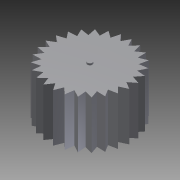
# Autodesk Inventor part: launcher.motor.lowgear
Saved by Autodesk Inventor 2011 (Build 150239000, 239)
## iProperties
Created: 2011-04-05
Part Number: launcher.motor.lowgear
Document SubType Name: Modeling
Designer: Rob
Density: 1 g/cm^3
Author: Rob
Autodesk Inventor part; units mm, degrees
ref_plane "YZ Plane" through (0, 0, 0) normal (1, 0, 0) x (0, 1, 0)
ref_plane "XZ Plane" through (0, 0, 0) normal (0, 1, 0) x (-1, 0, 0)
ref_plane "XY Plane" through (0, 0, 0) normal (0, 0, 1) x (1, 0, 0)
sketch "Sketch1" plane through (0, 0, 0) normal (0, 0, 1) x (1, 0, 0)
  circle A0 centre (0, 0) radius 2
  dimension "d0" = 4
  constraints: 1 centre point, 1 coincident
  measures "d0" diameter of A0
extrude "Extrusion1" add sketch "Sketch1" along normal blind 2.8
sketch "Sketch2" plane through (0, 0, 2.8) normal (0, 0, 1) x (1, 0, 0)
  circle A0 centre (0, 0) radius 0.5
  circle A1 centre (0, 0) radius 2
  line L0 (0, 0) -> (0, 5.155)
  line L1 (0, 2.4402) -> (-0.2438, 1.9851)
  line L2 (0, 2.4402) -> (0.2438, 1.9851)
  arc A2 (0.2438, 1.9851) -> (-0.2438, 1.9851) centre (0, 0) ccw
  line L3 (-0.2438, 1.9851) -> (0, 2.4402)
  line L4 (0, 2.4402) -> (0.2438, 1.9851)
  line L5 (-0.5628, 2.3745) -> (-0.695, 1.8754)
  line L6 (-0.5628, 2.3745) -> (-0.2206, 1.9878)
  arc A3 (-0.2206, 1.9878) -> (-0.695, 1.8754) centre (0, 0) ccw
  line L7 (-1.0952, 2.1807) -> (-1.1087, 1.6645)
  line L8 (-1.0952, 2.1807) -> (-0.6731, 1.8833)
  arc A4 (-0.6731, 1.8833) -> (-1.1087, 1.6645) centre (0, 0) ccw
  line L9 (-1.5686, 1.8693) -> (-1.4627, 1.364)
  line L10 (-1.5686, 1.8693) -> (-1.0893, 1.6774)
  arc A5 (-1.0893, 1.6774) -> (-1.4627, 1.364) centre (0, 0) ccw
  line L11 (-1.9574, 1.4572) -> (-1.7379, 0.9899)
  line L12 (-1.9574, 1.4572) -> (-1.4467, 1.3809)
  arc A6 (-1.4467, 1.3809) -> (-1.7379, 0.9899) centre (0, 0) ccw
  line L13 (-2.2407, 0.9665) -> (-1.9193, 0.5624)
  line L14 (-2.2407, 0.9665) -> (-1.7262, 1.0101)
  arc A7 (-1.7262, 1.0101) -> (-1.9193, 0.5624) centre (0, 0) ccw
  line L15 (-2.4032, 0.4237) -> (-1.9973, 0.1046)
  line L16 (-2.4032, 0.4237) -> (-1.9126, 0.5848)
  arc A8 (-1.9126, 0.5848) -> (-1.9973, 0.1046) centre (0, 0) ccw
  line L17 (-2.4361, -0.1419) -> (-1.9676, -0.3588)
  line L18 (-2.4361, -0.1419) -> (-1.9959, 0.1279)
  arc A9 (-1.9959, 0.1279) -> (-1.9676, -0.3588) centre (0, 0) ccw
  line L19 (-2.3377, -0.6999) -> (-1.8318, -0.8029)
  line L20 (-2.3377, -0.6999) -> (-1.9716, -0.3358)
  arc A10 (-1.9716, -0.3358) -> (-1.8318, -0.8029) centre (0, 0) ccw
  line L21 (-2.1133, -1.2201) -> (-1.5973, -1.2037)
  line L22 (-2.1133, -1.2201) -> (-1.841, -0.7814)
  arc A11 (-1.841, -0.7814) -> (-1.5973, -1.2037) centre (0, 0) ccw
  line L23 (-1.775, -1.6746) -> (-1.2766, -1.5396)
  line L24 (-1.775, -1.6746) -> (-1.6112, -1.1849)
  arc A12 (-1.6112, -1.1849) -> (-1.2766, -1.5396) centre (0, 0) ccw
  line L25 (-1.3409, -2.0388) -> (-0.8872, -1.7925)
  line L26 (-1.3409, -2.0388) -> (-1.2945, -1.5246)
  arc A13 (-1.2945, -1.5246) -> (-0.8872, -1.7925) centre (0, 0) ccw
  line L27 (-0.8346, -2.2931) -> (-0.4499, -1.9487)
  line L28 (-0.8346, -2.2931) -> (-0.908, -1.782)
  arc A14 (-0.908, -1.782) -> (-0.4499, -1.9487) centre (0, 0) ccw
  line L29 (-0.2833, -2.4237) -> (0.0117, -2)
  line L30 (-0.2833, -2.4237) -> (-0.4726, -1.9434)
  arc A15 (-0.4726, -1.9434) -> (0.0117, -2) centre (0, 0) ccw
  line L31 (0.2833, -2.4237) -> (0.4726, -1.9434)
  line L32 (0.2833, -2.4237) -> (-0.0117, -2)
  arc A16 (-0.0117, -2) -> (0.4726, -1.9434) centre (0, 0) ccw
  line L33 (0.8346, -2.2931) -> (0.908, -1.782)
  line L34 (0.8346, -2.2931) -> (0.4499, -1.9487)
  arc A17 (0.4499, -1.9487) -> (0.908, -1.782) centre (0, 0) ccw
  line L35 (1.3409, -2.0388) -> (1.2945, -1.5246)
  line L36 (1.3409, -2.0388) -> (0.8872, -1.7925)
  arc A18 (0.8872, -1.7925) -> (1.2945, -1.5246) centre (0, 0) ccw
  line L37 (1.775, -1.6746) -> (1.6112, -1.1849)
  line L38 (1.775, -1.6746) -> (1.2766, -1.5396)
  arc A19 (1.2766, -1.5396) -> (1.6112, -1.1849) centre (0, 0) ccw
  line L39 (2.1133, -1.2201) -> (1.841, -0.7814)
  line L40 (2.1133, -1.2201) -> (1.5973, -1.2037)
  arc A20 (1.5973, -1.2037) -> (1.841, -0.7814) centre (0, 0) ccw
  line L41 (2.3377, -0.6999) -> (1.9716, -0.3358)
  line L42 (2.3377, -0.6999) -> (1.8318, -0.8029)
  arc A21 (1.8318, -0.8029) -> (1.9716, -0.3358) centre (0, 0) ccw
  line L43 (2.4361, -0.1419) -> (1.9959, 0.1279)
  line L44 (2.4361, -0.1419) -> (1.9676, -0.3588)
  arc A22 (1.9676, -0.3588) -> (1.9959, 0.1279) centre (0, 0) ccw
  line L45 (2.4032, 0.4237) -> (1.9126, 0.5848)
  line L46 (2.4032, 0.4237) -> (1.9973, 0.1046)
  arc A23 (1.9973, 0.1046) -> (1.9126, 0.5848) centre (0, 0) ccw
  line L47 (2.2407, 0.9665) -> (1.7262, 1.0101)
  line L48 (2.2407, 0.9665) -> (1.9193, 0.5624)
  arc A24 (1.9193, 0.5624) -> (1.7262, 1.0101) centre (0, 0) ccw
  line L49 (1.9574, 1.4572) -> (1.4467, 1.3809)
  line L50 (1.9574, 1.4572) -> (1.7379, 0.9899)
  arc A25 (1.7379, 0.9899) -> (1.4467, 1.3809) centre (0, 0) ccw
  line L51 (1.5686, 1.8693) -> (1.0893, 1.6774)
  line L52 (1.5686, 1.8693) -> (1.4627, 1.364)
  arc A26 (1.4627, 1.364) -> (1.0893, 1.6774) centre (0, 0) ccw
  line L53 (1.0952, 2.1807) -> (0.6731, 1.8833)
  line L54 (1.0952, 2.1807) -> (1.1087, 1.6645)
  arc A27 (1.1087, 1.6645) -> (0.6731, 1.8833) centre (0, 0) ccw
  line L55 (0.5628, 2.3745) -> (0.2206, 1.9878)
  line L56 (0.5628, 2.3745) -> (0.695, 1.8754)
  arc A28 (0.695, 1.8754) -> (0.2206, 1.9878) centre (0, 0) ccw
  dimension "d5" = 360
  constraints: 114 end point, 54 point on circle, 28 centre point, 2 collinear, 1 point on line, 1 symmetric about line, 1 vertical, 193 other
extrude "Extrusion2" add sketch "Sketch2" against normal up to surface (2.8 mm away) contours A1 L6 L1 L0 | L0 L2 L55 A1 | L55 L2 A1 | A1 L1 L6 | L2 L55 L56 L53 A1 | A1 L8 L5 L6 L1 | L53 L56 A1 | A1 L5 L8 | L56 L53 L54 L51 A1 | A1 L10 L7 L8 L5 | L51 L54 A1 | A1 L7 L10 | L54 L51 L52 L49 A1 | A1 L12 L9 L10 L7 | L49 L52 A1 | A1 L9 L12 | L52 L49 L50 L47 A1 | A1 L14 L11 L12 L9 | L47 L50 A1 | A1 L11 L14 | L50 L47 L48 L45 A1 | A1 L16 L13 L14 L11 | L45 L48 A1 | A1 L13 L16 | L48 L45 L46 L43 A1 | A1 L18 L15 L16 L13 | L43 L46 A1 | A1 L15 L18 | L46 L43 L44 L41 A1 | A1 L20 L17 L18 L15 | A1 L17 L20 | L41 L44 A1 | L41 L42 L39 A1 L44 | A1 L22 L19 L20 L17 | A1 L19 L22 | L39 L42 A1 | L39 L40 L37 A1 L42 | A1 L24 L21 L22 L19 | A1 L21 L24 | L37 L40 A1 | L37 L38 L35 A1 L40 | A1 L26 L23 L24 L21 | A1 L23 L26 | L35 L38 A1 | L35 L36 L33 A1 L38 | A1 L28 L25 L26 L23 | A1 L25 L28 | L33 L36 A1 | L33 L34 L31 A1 L36 | A1 L30 L27 L28 L25 | A1 L27 L30 | L31 L34 A1 | L31 L32 L29 A1 L34 | A1 L32 L29 L30 L27 | A1 L29 L32
sketch "Sketch3" plane through (0, 0, 2.8) normal (0, 0, 1) x (1, 0, 0)
  circle A0 centre (0, 0) radius 0.1448
  constraints: 1 centre point, 1 coincident
extrude "Extrusion3" add sketch "Sketch3" along normal blind 0.1
body "Solid1"
